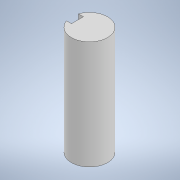
# Autodesk Inventor part: Shaft
Saved by Autodesk Inventor 2022 (Build 260153000, 153)
## iProperties
Created: 2022-08-20
Part Number: Shaft
Material: Generic
Document SubType Name: Modeling
Designer: Nick
Density: 1 g/cm^3
Appearance: Default
Mass: 7.42145 g
Surface Area: 26.3242 cm^2
Volume: 7.42145 cm^3
Author: Nick
Autodesk Inventor part; units mm, degrees
ref_plane "YZ Plane" through (0, 0, 0) normal (1, 0, 0) x (0, 1, 0)
ref_plane "XZ Plane" through (0, 0, 0) normal (0, 1, 0) x (-1, 0, 0)
ref_plane "XY Plane" through (0, 0, 0) normal (0, 0, 1) x (1, 0, 0)
sketch "Sketch1" plane through (0, 0, 0) normal (0, 1, 0) x (-1, 0, 0)
  circle A0 centre (0, 0) radius 7.5
  line L0 (10, 2.5) -> (5, 2.5)
  line L1 (5, 2.5) -> (5, -2.5)
  line L2 (5, -2.5) -> (10, -2.5)
  line L3 (10, -2.5) -> (10, 2.5)
  point P0 (7.5, 0)
  point P1 (7.5, -2.5)
  point P2 (5, 0)
  point P3 (7.0711, 2.5)
  point P4 (7.0711, -2.5)
  dimension "d0" = 15
  dimension "d1" = 5
  dimension "d2" = 5
  constraints: 8 end point, 2 horizontal alignment, 2 midpoint, 2 parallel, 1 coincident, 1 horizontal, 1 perpendicular, 1 vertical alignment, 3 other
  measures "d1" distance of L2.end L1.end
  measures "d2" distance of L1.end L0.end
extrude "Extrusion1" add sketch "Sketch1" along normal blind 45 contours L0 L1 L2 A0 picked at (0.8519, -0.3038)
body "Solid1"
